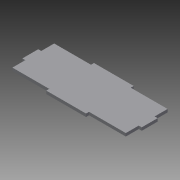
# Autodesk Inventor part: Top
Saved by Autodesk Inventor 2013 (Build 170138000, 138)
## iProperties
Created: 2013-04-20
Part Number: Top
Material: Generic
Document SubType Name: Modeling
Designer: fuji
Density: 1 g/cm^3
Author: fuji
Autodesk Inventor part; units mm, degrees
ref_plane "YZ Plane" through (0, 0, 0) normal (1, 0, 0) x (0, 1, 0)
ref_plane "XZ Plane" through (0, 0, 0) normal (0, 1, 0) x (-1, 0, 0)
ref_plane "XY Plane" through (0, 0, 0) normal (0, 0, 1) x (1, 0, 0)
sketch "Sketch1" plane through (0, 0, 0) normal (0, 1, 0) x (-1, 0, 0)
  line L0 (0, 0) -> (120.65, 0)
  line L1 (120.65, 0) -> (120.65, 44.45)
  line L2 (120.65, 44.45) -> (0, 44.45)
  line L3 (0, 44.45) -> (0, 0)
  dimension "d0" = 120.65
  dimension "d1" = 44.45
  constraints: 8 end point, 2 parallel, 1 horizontal, 1 perpendicular
  measures "d0" distance of L2.end L1.end
  measures "d1" distance of L1.end L0.end
extrude "Extrusion1" add sketch "Sketch1" along normal blind 3.175
sketch "Sketch2" plane through (0, 3.175, 0) normal (0, 1, 0) x (1, 0, 0)
  line L0 (0, 0) -> (-120.65, 0) projected
  line L1 (-120.65, 0) -> (-120.65, -44.45) projected
  line L2 (-120.65, -44.45) -> (0, -44.45) projected
  line L3 (0, -44.45) -> (0, 0) projected
  line L4 (-81.4917, 0) -> (-39.1583, 0)
  line L5 (-39.1583, 0) -> (-39.1583, 3.175)
  line L6 (-39.1583, 3.175) -> (-81.4917, 3.175)
  line L7 (-81.4917, 3.175) -> (-81.4917, 0)
  line L8 (-81.4917, -44.45) -> (-39.1583, -44.45)
  line L9 (-39.1583, -44.45) -> (-39.1583, -47.625)
  line L10 (-39.1583, -47.625) -> (-81.4917, -47.625)
  line L11 (-81.4917, -47.625) -> (-81.4917, -44.45)
  line L12 (0, -13.7583) -> (3.175, -13.7583)
  line L13 (3.175, -13.7583) -> (3.175, -30.6917)
  line L14 (3.175, -30.6917) -> (0, -30.6917)
  line L15 (0, -30.6917) -> (0, -13.7583)
  line L16 (-120.65, -13.7583) -> (-123.825, -13.7583)
  line L17 (-123.825, -13.7583) -> (-123.825, -30.6917)
  line L18 (-123.825, -30.6917) -> (-120.65, -30.6917)
  line L19 (-120.65, -30.6917) -> (-120.65, -13.7583)
  dimension "d4" = 42.3333
  dimension "d5" = 3.175
  dimension "d6" = 39.1583
  dimension "d7" = 42.3333
  dimension "d8" = 3.175
  dimension "d9" = 3.175
  dimension "d10" = 16.9333
  dimension "d11" = 3.175
  dimension "d12" = 16.9333
  dimension "d13" = 13.7583
  constraints: 32 end point, 8 parallel, 4 horizontal, 4 perpendicular, 4 point on line, 2 collinear
  measures "d4" distance of L6.end L5.end
  measures "d5" distance of L5.end L4.end
  measures "d6" distance between parallel lines of L7 L1
  measures "d7" distance of L9.end L10.end
  measures "d8" distance of L8.end L9.end
  measures "d9" distance of L13.end L14.end
  measures "d10" distance of L12.end L13.end
  measures "d11" distance of L18.end L17.end
  measures "d12" distance of L17.end L16.end
  measures "d13" distance between parallel lines of L16 L0
extrude "Extrusion2" add sketch "Sketch2" against normal blind 3.175 contours L0 L7 L6 L5 | L12 L13 L14 L3 | L1 L18 L17 L16 | L9 L10 L11 L2
equation "\"d0\" = width - 2 * thick"
equation "\"d1\" = depth - 2 * thick"
equation "\"d2\" = thick"
equation "\"d4\" = 0.333333 * width"
equation "\"d5\" = thick"
equation "\"d6\" = 0.333333 * width - thick"
equation "\"d7\" = 0.333333 * width"
equation "\"d8\" = thick"
equation "\"d9\" = thick"
equation "\"d10\" = 0.333333 * depth"
equation "\"d11\" = thick"
equation "\"d12\" = 0.333333 * depth"
equation "\"d13\" = 0.333333 * depth - thick"
equation "\"d14\" = thick"
equation "\"width\" = 127"
equation "\"thick\" = 3.175"
equation "\"depth\" = 50.8"
body "Solid1"
